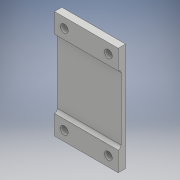
# Autodesk Inventor part: piston-mount
Saved by Autodesk Inventor 2018 (Build 220112000, 112)
## iProperties
Created: 2025-02-25
Part Number: piston-mount
Material: Generic
Document SubType Name: Modeling
Designer: neo
Density: 1 g/cm^3
Appearance: Default
Author: neo
Autodesk Inventor part; units mm, degrees
ref_plane "YZ Plane" through (0, 0, 0) normal (1, 0, 0) x (0, 1, 0)
ref_plane "XZ Plane" through (0, 0, 0) normal (0, 1, 0) x (-1, 0, 0)
ref_plane "XY Plane" through (0, 0, 0) normal (0, 0, 1) x (1, 0, 0)
sketch "Sketch1" plane through (0, 0, 0) normal (0, 1, 0) x (-1, 0, 0)
  circle A0 centre (9, 18) radius 1.6
  line L0 (0, 26.5631) -> (0, -32.5504)
  line L1 (19.3723, 0) -> (-25.4899, 0)
  circle A1 centre (9, -18) radius 1.6
  circle A2 centre (-9, 18) radius 1.6
  circle A3 centre (-9, -18) radius 1.6
  line L2 (13, 22) -> (-13, 22)
  line L3 (-13, 22) -> (-13, -22)
  line L4 (-13, -22) -> (13, -22)
  line L5 (13, -22) -> (13, 22)
  point P0 (0, 0)
  dimension "d0" = 3.2
  dimension "d3" = 36
  dimension "d6" = 18
  dimension "d9" = 4
  dimension "d10" = 4
  constraints: 12 end point, 4 centre point, 3 horizontal, 2 parallel, 2 vertical, 1 perpendicular, 10 other
  measures "d0" diameter of A0
  measures "d3" distance of A0.centre A1.centre
  measures "d6" distance of A0.centre A2.centre
  measures "d9" distance from line of L2 A0.centre
  measures "d10" distance from line of L5 A0.centre
extrude "Extrusion1" add sketch "Sketch1" along normal blind 3
sketch "Sketch2" plane through (13, 0, 22) normal (1, 0, 0) x (0, 0, -1)
  line L0 (0, 0) -> (44, 0) projected
  line L1 (44, 0) -> (44, 3) projected
  line L2 (0, 3) -> (44, 3) projected
  line L3 (0, 0) -> (0, 3) projected
  line L4 (0, 0) -> (44, 0) projected
  line L5 (8, 1.2) -> (36, 1.2)
  line L6 (36, 1.2) -> (36, 0)
  line L7 (36, 0) -> (8, 0)
  line L8 (8, 0) -> (8, 1.2)
  point P0 (22, 0)
  dimension "d13" = 1.2
  dimension "w" = 8
  dimension "d15" = 8
  constraints: 8 end point, 2 parallel, 1 horizontal, 1 perpendicular, 1 point on line
  measures "d13" distance between parallel lines of L0 L5
  measures "w" distance between parallel lines of L3 L8
  measures "d15" distance between parallel lines of L1 L6
extrude "Extrusion2" cut sketch "Sketch2" against normal through all contours L8 L5 L6 L0
fillet "Fillet1" radius 1.2 2 edges at (0, 1.2, -14) (0, 1.2, 14)
equation "\"d15\" = w"
body "Solid1"
